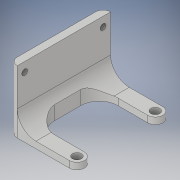
# Autodesk Inventor part: pi_camera_mount
Saved by Autodesk Inventor 2019 (Build 230136000, 136)
## iProperties
Created: 2020-10-08
Part Number: pi_camera_mount
Material: Generic
Document SubType Name: Modeling
Designer: infinity
Density: 1 g/cm^3
Appearance: Default
Author: infinity
Autodesk Inventor part; units mm, degrees
ref_plane "YZ Plane" through (0, 0, 0) normal (1, 0, 0) x (0, 1, 0)
ref_plane "XZ Plane" through (0, 0, 0) normal (0, 1, 0) x (-1, 0, 0)
ref_plane "XY Plane" through (0, 0, 0) normal (0, 0, 1) x (1, 0, 0)
sketch "Sketch1" plane through (0, 0, 0) normal (0, 1, 0) x (-1, 0, 0)
  line L0 (0, 0) -> (0, 0)
  line L1 (0, -2) -> (0, -23)
  line L2 (0, -25) -> (-1.1394, -25)
  line L3 (-3, -16) -> (-3, -9)
  line L4 (-2, 0) -> (-16, 0)
  line L5 (-18, -2) -> (-18, -2)
  line L6 (-16, -4) -> (-8, -4)
  line L7 (-2, -25) -> (-16, -25)
  line L8 (-18, -23) -> (-18, -23)
  line L9 (-16, -21) -> (-8, -21)
  arc A0 (-3, -9) -> (-8, -4) centre (-8, -9) ccw
  arc A1 (-8, -21) -> (-3, -16) centre (-8, -16) ccw
  arc A2 (-16, 0) -> (-18, -2) centre (-16, -2) ccw
  arc A3 (-18, -2) -> (-16, -4) centre (-16, -2) ccw
  arc A4 (-16, -21) -> (-18, -23) centre (-16, -23) ccw
  arc A5 (-18, -23) -> (-16, -25) centre (-16, -23) ccw
  arc A6 (0, -2) -> (-2, 0) centre (-2, -2) ccw
  arc A7 (-2, -25) -> (0, -23) centre (-2, -23) ccw
  point P0 (-18, -21)
  point P1 (-18, -25)
  point P2 (-16, -2)
  point P3 (-16, -23)
  dimension "d0" = 3
  dimension "d2" = 4
  dimension "d3" = 2
  dimension "d4" = 2
  dimension "d5" = 2
  dimension "d6" = 2
  dimension "d7" = 4
  dimension "d8" = 21
  dimension "d9" = 15
  dimension "d10" = 0
  dimension "d11" = 5
  dimension "d12" = 2
  constraints: 20 end point, 16 point on circle, 16 tangent, 9 point on line, 8 centre point, 6 equal radius, 4 parallel, 3 horizontal, 3 perpendicular
  measures "d0" distance between parallel lines of L3 L1
  measures "d2" distance between parallel lines of L6 L4
  measures "d3" distance from line of L6 point (-16, -2)
  measures "d4" distance from line of point (-16, -2) L5
  measures "d5" distance from line of L8 point (-16, -23)
  measures "d6" distance from line of L7 point (-16, -23)
  measures "d7" distance of point (-18, -25) point (-18, -21)
  measures "d8" distance of point (-16, -23) point (-16, -2)
  measures "d9" distance between parallel lines of L8 L3
  measures "d10" distance from line of L0.start L1
  measures "d11" radius of A0
  measures "d12" radius of A2
extrude "Extrusion1" add sketch "Sketch1" along normal blind 1.75
sketch "Sketch2" plane through (0, 1.75, 0) normal (0, 1, 0) x (1, 0, 0)
  arc A0 (0, 2) -> (2, 0) centre (2, 2) ccw projected
  line L0 (0, 23) -> (0, 2) projected
  arc A1 (2, 25) -> (0, 23) centre (2, 23) ccw projected
  line L1 (2, 0) -> (2, 25)
  point P0 (0, 0)
  constraints: 2 end point, 1 vertical
extrude "Extrusion2" add sketch "Sketch2" along normal blind 15
hole "Hole1" at (16, 0, -2) at (16, 0, -23) direction (0, 1, 0) diameter 2.4 depth 6.3 tip angle 118 clearance for "Flat Head Machine Screw" size "M2" standard "Ansi Metric M Profile"
fillet "Fillet1" radius 5 1 edges at (2, 1.75, -12.5)
sketch "Sketch3" plane through (2, 16.75, 0) normal (1, 0, 0) x (0, 0, -1)
  line L0 (2, -2.5) -> (23, -2.5) construction
  line L1 (25, -10) -> (25, 0) projected
  line L2 (0, -10) -> (0, 0) projected
  line L3 (0, 0) -> (25, 0) projected
  point P0 (0, -16.75)
  dimension "d25" = 21
  dimension "d26" = 25
  dimension "d27" = 2
  dimension "d28" = 2.5
  constraints: 2 coincident, 2 end point
  measures "d25" distance of L0.start L0.end
  measures "d26" distance between parallel lines of L1 L2
  measures "d27" distance from line of L0.start L2
  measures "d28" distance between parallel lines of L0 L3
hole "Hole2" at (2, 14.25, -2) at (2, 14.25, -23) direction (-1, 0, 0) diameter 1.567 depth 6.3 tip angle 118 thread size "M2x0.4" class "6H" standard "ANSI Metric M Profile"
equation "\"d3\" = 0.5 * d2"
equation "\"d4\" = d3"
equation "\"d5\" = d3"
equation "\"d6\" = d4"
equation "\"d7\" = d2"
equation "\"d27\" = -0.5 * d25 + 0.5 * d26"
body "Solid1"
